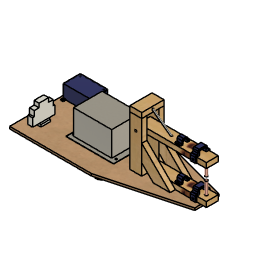
MOT Welder (Autodesk Fusion 360 design; units mm, degrees)
Autodesk Fusion 360 part; units mm, degrees
sketch "Sketch1" plane through (0, 0, 0) normal (0, 0, 1) x (1, 0, 0)
  line L0 (0, 0) -> (600, 0)
  line L1 (600, 0) -> (600, -250)
  line L2 (600, -250) -> (0, -250)
  line L3 (0, -250) -> (0, 0)
  line L4 (300, -250) -> (600, -169.6152)
  line L5 (300, -250) -> (610.5829, -250) construction
  line L6 (300, 0) -> (600, -80.3848)
  dimension "d1" = 600
  dimension "d2" = 250
  dimension "d104" = 15
  dimension "d105" = 15
  constraint horizontal L0
  constraint vertical L1
  constraint horizontal L2
  constraint vertical L3
  constraint coincident L0.start L3.end
  constraint horizontal L5
  constraint midpoint L2 L4.start
  constraint coincident L1 L4.end
  constraint midpoint L0 L6.start
  constraint coincident L1 L6.end
  measures "d1" distance of L1.end L2.end
  measures "d2" distance of L0.start L2.end
  measures "d104" angle of L4 L5
  measures "d105" angle of L0 L6
extrude "Extrude1" add sketch "Sketch1" against normal blind 8 contours L0 L1 L2 L3 L4 L6 makes body 1
sketch "Sketch2" plane through (0, 0, 0) normal (0, 0, 1) x (-1, 0, 0)
  line L0 (0, 250) -> (-300, 250)
  line L1 (-600, 169.6152) -> (-600, 80.3848)
  line L2 (-300, 0) -> (0, 0)
  line L3 (0, 0) -> (0, 250)
  line L4 (0, 0) -> (-150, 0)
  line L5 (-150, 0) -> (-150, 60)
  line L6 (-150, 60) -> (0, 60)
  line L7 (0, 60) -> (0, 0)
  line L8 (-150, 60) -> (-290, 60)
  line L9 (-290, 60) -> (-290, 165)
  line L10 (-290, 165) -> (-150, 165)
  line L11 (-150, 165) -> (-150, 60)
  line L12 (-136, 165) -> (-136, 60)
  line L13 (-290, 179) -> (-150, 179)
  line L14 (-311, 60) -> (-311, 165)
  line L15 (-136, 165) -> (-136, 179)
  line L16 (-136, 179) -> (-150, 179)
  line L17 (-311, 165) -> (-311, 179)
  line L18 (-311, 179) -> (-290, 179)
  line L19 (-311, 60) -> (-290, 60)
  line L20 (-136, 60) -> (-143, 60)
  line L21 (-143, 60) -> (-143, 70)
  line L22 (-143, 70) -> (-136, 70)
  line L23 (-136, 70) -> (-136, 60)
  line L24 (-136, 179) -> (-143, 179)
  line L25 (-143, 179) -> (-143, 159)
  line L26 (-143, 159) -> (-136, 159)
  line L27 (-136, 159) -> (-136, 179)
  line L28 (-311, 60) -> (-300.5, 60)
  line L29 (-300.5, 60) -> (-300.5, 70)
  line L30 (-300.5, 70) -> (-311, 70)
  line L31 (-311, 70) -> (-311, 60)
  line L32 (-311, 179) -> (-300.5, 179)
  line L33 (-300.5, 179) -> (-300.5, 159)
  line L34 (-300.5, 159) -> (-311, 159)
  line L35 (-311, 159) -> (-311, 179)
  circle A0 centre (-143, 70) radius 3
  circle A1 centre (-300.5, 70) radius 3
  circle A2 centre (-300.5, 159) radius 3
  circle A3 centre (-143, 159) radius 3
  line L36 (-300, 250) -> (-600, 169.6152)
  line L37 (-600, 80.3848) -> (-300, 0)
  dimension "d5" = 140
  dimension "d6" = 105
  dimension "d7" = -14
  dimension "d8" = -14
  dimension "d9" = -21
  dimension "d14" = 7
  dimension "d15" = 10
  dimension "d16" = 7
  dimension "d17" = 20
  dimension "d18" = 10
  dimension "d19" = 20
  dimension "d20" = 6
  dimension "d21" = 6
  dimension "d22" = 6
  dimension "d23" = 6
  dimension "d24" = 10.5
  dimension "d25" = 10.5
  dimension "d26" = 150
  dimension "d27" = 60
  constraint horizontal L4
  constraint vertical L5
  constraint horizontal L6
  constraint vertical L7
  constraint coincident L2.end L3.start
  constraint horizontal L8
  constraint vertical L9
  constraint horizontal L10
  constraint vertical L11
  constraint perpendicular L13 L15
  constraint perpendicular L15 L16
  constraint perpendicular L13 L17
  constraint perpendicular L17 L18
  constraint perpendicular L9 L19
  constraint horizontal L20
  constraint vertical L21
  constraint horizontal L22
  constraint vertical L23
  constraint horizontal L24
  constraint vertical L25
  constraint horizontal L26
  constraint vertical L27
  constraint horizontal L28
  constraint vertical L29
  constraint horizontal L30
  constraint vertical L31
  constraint horizontal L32
  constraint vertical L33
  constraint horizontal L34
  constraint vertical L35
  constraint coincident L21.end L22.start
  constraint coincident L29.end L30.start
  constraint coincident L33.end L34.start
  constraint coincident L25.end L26.start
  measures "d5" distance of L5.end L8.end
  measures "d6" distance of L5.end L10.end
  measures "d14" distance of L12.end L20.end
  measures "d15" distance of L12.end L22.end
  measures "d16" distance of L15.end L24.end
  measures "d17" distance of L15.end L26.end
  measures "d18" distance of L14.start L30.end
  measures "d19" distance of L17.end L34.end
  measures "d20" diameter of A0
  measures "d21" diameter of A1
  measures "d22" diameter of A2
  measures "d23" diameter of A3
  measures "d24" distance of L29.end L30.end
  measures "d25" distance of L33.end L34.end
  measures "d26" distance of L5.end L6.end
  measures "d27" distance of L4.end L5.end
extrude "Extrude2" add sketch "Sketch2" along normal blind 1 separate body contours L6 L12 L20 L21 L22 L23 A0 | L6 L9 L10 L11 L12 L13 L14 L16 L18 L19 L21 L22 L25 L26 L29 L30 L33 L34 A0 A1 A2 A3 | L12 L15 L16 L24 L25 L26 L27 A3 | L14 L19 L28 L29 L30 L31 A1 | L14 L17 L18 L32 L33 L34 L35 A2 makes body 2
extrude "Extrude3" add sketch "Sketch2" along normal blind 92 separate body contours L8 L9 L10 L11 makes body 3
combine "Combine2" operation add target body 3 tool bodies 2
ref_plane "WorkPlane1" through (370, -112.5, 46) normal (1, 0, 0) x (0, 1, 0)
sketch "Sketch3" plane through (370, 0, 0) normal (1, 0, 0) x (0, 1, 0)
  line L0 (0, 0) -> (-250, 0)
  line L1 (-125, 0) -> (-125, 9.5)
  line L2 (-103, 0) -> (-147, 0)
  line L3 (-147, 0) -> (-147, 19)
  line L4 (-147, 19) -> (-103, 19)
  line L5 (-103, 19) -> (-103, 0)
  line L6 (-103, 0) -> (-147, 19) construction
  line L7 (-147, 0) -> (-103, 19) construction
  line L8 (-125, 19) -> (-125, 124)
  line L9 (-125, 124) -> (-125, 133.5)
  line L10 (-103, 124) -> (-147, 124)
  line L11 (-147, 124) -> (-147, 143)
  line L12 (-147, 143) -> (-103, 143)
  line L13 (-103, 143) -> (-103, 124)
  line L14 (-103, 124) -> (-147, 143) construction
  line L15 (-147, 124) -> (-103, 143) construction
  point P0 (-125, 9.5)
  point P1 (-125, 133.5)
  dimension "d29" = 250
  dimension "d30" = 9.5
  dimension "d31" = 44
  dimension "d32" = 105
  dimension "d33" = 9.5
  dimension "d34" = 44
  dimension "d35" = 19
  constraint coincident L0.start origin
  constraint horizontal L0
  constraint midpoint L0 L1.start
  constraint perpendicular L0 L1
  constraint horizontal L2
  constraint perpendicular L2 L3
  constraint parallel L2 L4
  constraint parallel L3 L5
  constraint coincident L6 P0
  constraint coincident L7 P0
  constraint coincident P0 L1.end
  constraint midpoint L4 L8.start
  constraint perpendicular L4 L8
  constraint vertical L9
  constraint horizontal L10
  constraint perpendicular L10 L11
  constraint parallel L10 L12
  constraint parallel L11 L13
  constraint coincident L14 P1
  constraint coincident L15 P1
  constraint coincident P1 L9.end
  measures "d29" distance of L0.start L0.end
  measures "d30" distance of L1.start P0
  measures "d31" distance of L3.end L4.end
  measures "d32" distance of L8.start L8.end
  measures "d33" distance of L8.end P1
  measures "d34" distance of L11.end L12.end
  measures "d35" distance of L10.end L11.end
extrude "Extrude4" add sketch "Sketch3" along normal blind 250 separate body makes body 4 at (453.3333, -117.6667, 124) makes body 5 at (453.3333, -117.6667, 0)
sketch "Sketch5" plane through (0, -103, 0) normal (0, 1, 0) x (-1, 0, 0)
  line L0 (-370, 124) -> (-370, 143)
  line L1 (-370, 143) -> (-620, 143)
  line L2 (-620, 143) -> (-620, 124)
  line L3 (-620, 124) -> (-370, 124)
  line L4 (-370, 124) -> (-379.5, 124)
  line L5 (-379.5, 124) -> (-379.5, 133.5)
  line L6 (-379.5, 133.5) -> (-370, 133.5)
  line L7 (-370, 133.5) -> (-370, 124)
  circle A0 centre (-379.5, 133.5) radius 4
  circle A1 centre (-379.5, 133.5) radius 11
  line L8 (-357.5, 183.5) -> (-401.5, 183.5)
  line L9 (-401.5, 183.5) -> (-401.5, 83.5)
  line L10 (-401.5, 83.5) -> (-357.5, 83.5)
  line L11 (-357.5, 83.5) -> (-357.5, 183.5)
  line L12 (-357.5, 183.5) -> (-401.5, 83.5) construction
  line L13 (-401.5, 183.5) -> (-357.5, 83.5) construction
  line L14 (-401.5, 83.5) -> (-357.5, 83.5)
  line L15 (-357.5, 83.5) -> (-357.5, 0)
  line L16 (-357.5, 0) -> (-401.5, 0)
  line L17 (-401.5, 0) -> (-401.5, 83.5)
  line L18 (-401.5, 0) -> (-422.7132, 21.2132)
  line L19 (-401.5, 0) -> (-357.5, 0) construction
  line L20 (-422.7132, 21.2132) -> (-401.5, 42.4264)
  line L21 (-422.7132, 21.2132) -> (-443.9264, 0)
  line L22 (-401.5, 0) -> (-443.9264, 0)
  line L23 (-453.8259, 52.3259) -> (-475.0391, 31.1127)
  line L24 (-453.8259, 52.3259) -> (-432.6127, 73.5391)
  line L25 (-443.9264, 0) -> (-506.1518, 0)
  line L26 (-506.1518, 0) -> (-475.0391, 31.1127)
  line L27 (-432.6127, 73.5391) -> (-401.5, 104.6518)
  point P0 (-379.5, 133.5)
  dimension "d38" = 9.5
  dimension "d39" = 9.5
  dimension "d40" = 8
  dimension "d41" = 22
  dimension "d42" = 44
  dimension "d43" = 100
  dimension "d44" = 44
  dimension "d45" = 83.5
  dimension "d57" = 135
  dimension "d58" = 30
  dimension "d59" = -44
  constraint horizontal L4
  constraint vertical L5
  constraint horizontal L6
  constraint vertical L7
  constraint coincident L0.start L3.end
  constraint coincident P0 L5.end
  constraint concentric A0 A1
  constraint horizontal L8
  constraint perpendicular L8 L9
  constraint parallel L8 L10
  constraint parallel L9 L11
  constraint coincident L12 P0
  constraint coincident L13 P0
  constraint horizontal L14
  constraint vertical L15
  constraint horizontal L16
  constraint vertical L17
  constraint horizontal L19
  constraint coincident L17 L20.end
  constraint perpendicular L18 L20
  constraint perpendicular L18 L21
  constraint perpendicular L17 L22
  constraint parallel L22 L25
  constraint parallel L23 L26
  constraint coincident L17 L27.end
  constraint parallel L24 L27
  measures "d38" distance of L0.start L4.end
  measures "d39" distance of L0.start L6.end
  measures "d40" diameter of A0
  measures "d41" diameter of A1
  measures "d42" distance of L9.end L10.end
  measures "d43" distance of L8.end L9.end
  measures "d44" distance of L9.end L10.end
  measures "d45" distance of L9.end L16.end
  measures "d57" angle of L18 L19
  measures "d58" distance of L16.end L18.end
extrude "Extrude5" add sketch "Sketch5" along normal blind 19 separate body contours L0 L3 L4 L7 A1 | L0 L1 L3 L4 L7 A1 L8 L9 L10 L11 L14 | L0 L3 L4 L5 L6 L7 A0 A1 | L0 L7 A1 | L3 L4 A1 | L0 L1 L3 L5 L6 A0 A1 | L1 L3 A1 L9 | L0 L1 A1 | L1 A1 | L10 L14 L15 L16 L17 makes body 6
extrude "Extrude6" cut sketch "Sketch5" along normal blind 7 contours L0 L3 L4 L5 L6 L7 A0 A1 | L0 L7 A1 | L3 L4 A1 | L0 L1 L3 L5 L6 A0 A1 | L1 A1 bodies 6
extrude "Extrude8" add sketch "Sketch5" along normal blind 19 separate body contours L9 L17 L20 L21 L23 L24 L25 L26 L27 makes body 7
ref_plane "WorkPlane2" through (495, -125, 133.5) normal (0, 1, 0) x (0, 0, 1)
mirror "Mirror1" about plane through (495, -125, 133.5) normal (0, 1, 0) of bodies 7 6 makes body 8 at (379.4004, -166, 43.1704) makes body 9 at (475.0391, -147, 10.3709)
sketch "Sketch6" plane through (0, 0, 183.5) normal (0, 0, 1) x (-1, 0, 0)
  line L0 (-357.5, 103) -> (-401.5, 103)
  line L1 (-401.5, 103) -> (-401.5, 84)
  line L2 (-401.5, 84) -> (-357.5, 84)
  line L3 (-357.5, 84) -> (-357.5, 103)
  line L4 (-357.5, 84) -> (-401.5, 84)
  line L5 (-401.5, 84) -> (-401.5, 166)
  line L6 (-401.5, 166) -> (-357.5, 166)
  line L7 (-357.5, 166) -> (-357.5, 84)
  dimension "d53" = 44
  dimension "d54" = 82
  constraint horizontal L4
  constraint vertical L5
  constraint horizontal L6
  constraint vertical L7
  constraint coincident L2.end L3.start
  measures "d53" distance of L2.end L1.end
  measures "d54" distance of L2.end L6.end
extrude "Extrude7" add sketch "Sketch6" along normal blind 19 separate body makes body 10
sketch "Sketch7" plane through (0, 0, -8) normal (0, 0, -1) x (1, 0, 0)
  line L0 (300, 250) -> (0, 250)
  line L1 (0, 250) -> (0, 0)
  line L2 (0, 0) -> (300, 0)
  line L3 (600, 80.3848) -> (600, 169.6152)
  line L4 (0, 250) -> (40, 250)
  line L5 (40, 250) -> (40, 210)
  line L6 (40, 210) -> (0, 210)
  line L7 (0, 210) -> (0, 250)
  circle A0 centre (40, 210) radius 21.5
  circle A1 centre (40, 210) radius 29
  line L8 (600, 169.6152) -> (300, 250)
  line L9 (300, 0) -> (600, 80.3848)
  dimension "d62" = 40
  dimension "d63" = 40
  dimension "d64" = 43
  dimension "d65" = 58
  constraint horizontal L4
  constraint vertical L5
  constraint horizontal L6
  constraint vertical L7
  constraint coincident L0.end L1.start
  constraint coincident L5.end L6.start
  constraint concentric A0 A1
  measures "d62" distance of L0.end L4.end
  measures "d63" distance of L0.end L6.end
  measures "d64" diameter of A0
  measures "d65" diameter of A1
extrude "Extrude9" add sketch "Sketch7" along normal blind 20 separate body contours L5 L6 A0 | L5 L6 A0 makes body 11
loft "Loft1" add profiles "Sketch7" section 1 contours L5 L6 A0 A1 | L5 L6 A0 A1 section 2 face at (46.6953, -203.71, -28) separate body on bodies 11 makes body 12
combine "Combine1" operation add target body 11 tool bodies 12
fillet "Fillet1" radius 5 1 edges at (19.955, -202.2253, -28) on bodies 11
pattern_linear "R-Pattern1" count 2 spacing 170 along (0, 1, 0) count 2 spacing 260 along (1, 0, 0) of bodies 11 makes body 13 at (44.1141, -67.2954, -11.7235) makes body 14 at (304.1141, -237.2954, -11.7235) makes body 15 at (304.1141, -67.2954, -11.7235)
sketch "Sketch8" plane through (0, 0, 124) normal (0, 0, -1) x (1, 0, 0)
  line L0 (370, 147) -> (370, 103)
  line L1 (370, 103) -> (620, 103)
  line L2 (620, 103) -> (620, 147)
  line L3 (620, 147) -> (370, 147)
  line L4 (620, 147) -> (598, 147)
  line L5 (598, 147) -> (598, 125)
  line L6 (598, 125) -> (620, 125)
  line L7 (620, 125) -> (620, 147)
  circle A0 centre (598, 125) radius 5
  dimension "d74" = 22
  dimension "d75" = 10
  constraint horizontal L4
  constraint vertical L5
  constraint horizontal L6
  constraint vertical L7
  constraint coincident L2.end L3.start
  constraint coincident L5.end L6.start
  measures "d74" distance of L2.end L4.end
  measures "d75" diameter of A0
extrude "Extrude10" add sketch "Sketch8" along normal blind 105 separate body contours L5 L6 A0 | L5 L6 A0 makes body 16
extrude "Extrude11" cut 1 faces at (599.0448, -126.4407, 124) along direction (0, 0, -1) blind 54.5 on bodies 16 bodies 16
extrude "Extrude12" add sketch "Sketch8" along normal blind 50.5 separate body contours L5 L6 A0 | L5 L6 A0 makes body 17
chamfer "Chamfer1" distance 5 angle 45 2 edges at (593.3384, -123.1919, 69.5) (593.3384, -123.1919, 73.5) on bodies 16 17
sketch "Sketch9" plane through (401.5, 0, 0) normal (1, 0, 0) x (0, 1, 0)
  line L0 (-166, 183.5) -> (-84, 183.5)
  line L1 (-84, 183.5) -> (-84, 202.5)
  line L2 (-84, 202.5) -> (-166, 202.5)
  line L3 (-166, 202.5) -> (-166, 183.5)
  line L4 (-125, 202.5) -> (-125, 193)
  circle A0 centre (-125, 193) radius 3.5
  dimension "d83" = 9.5
  dimension "d84" = 7
  constraint midpoint L2 L4.start
  constraint perpendicular L2 L4
  constraint coincident L4.end A0.centre
  measures "d83" distance of L4.start L4.end
  measures "d84" diameter of A0
sketch "Sketch10" plane through (0, 0, 143) normal (0, 0, 1) x (-1, 0, 0)
  line L0 (-370, 103) -> (-370, 147)
  line L1 (-370, 147) -> (-620, 147)
  line L2 (-620, 147) -> (-620, 103)
  line L3 (-620, 103) -> (-370, 103)
  line L4 (-370, 125) -> (-470, 125)
  circle A0 centre (-470, 125) radius 3.5
  dimension "d85" = 100
  dimension "d86" = 7
  constraint midpoint L0 L4.start
  constraint perpendicular L0 L4
  constraint coincident L4.end A0.centre
  measures "d85" distance of L4.start L4.end
  measures "d86" diameter of A0
loft "Loft2" add profiles "Sketch10", "Sketch9" section 1 contours A0 section 2 contours A0 separate body makes body 18
sketch "Sketch11" plane through (0, 0, 0) normal (0, 0, 1) x (-1, 0, 0)
  line L0 (0, 250) -> (-300, 250)
  line L1 (-600, 169.6152) -> (-600, 80.3848)
  line L2 (-300, 0) -> (0, 0)
  line L3 (0, 0) -> (0, 250)
  line L4 (0, 0) -> (-30, 0)
  line L5 (-30, 0) -> (-30, 160)
  line L6 (-30, 160) -> (0, 160)
  line L7 (0, 160) -> (0, 0)
  line L8 (-30, 160) -> (-60, 160)
  line L9 (-60, 160) -> (-60, 195)
  line L10 (-60, 195) -> (-30, 195)
  line L11 (-30, 195) -> (-30, 160)
  line L12 (-300, 250) -> (-600, 169.6152)
  line L13 (-600, 80.3848) -> (-300, 0)
  dimension "d87" = 30
  dimension "d88" = 160
  dimension "d89" = 30
  dimension "d90" = 35
  constraint horizontal L4
  constraint vertical L5
  constraint horizontal L6
  constraint vertical L7
  constraint coincident L2.end L3.start
  constraint horizontal L8
  constraint vertical L9
  constraint horizontal L10
  constraint vertical L11
  measures "d87" distance of L2.end L4.end
  measures "d88" distance of L2.end L6.end
  measures "d89" distance of L5.end L8.end
  measures "d90" distance of L5.end L10.end
extrude "Extrude13" add sketch "Sketch11" along normal blind 8 separate body contours L8 L9 L10 L11 makes body 19
sketch "Sketch12" plane through (0, 0, 8) normal (0, 0, 1) x (-1, 0, 0)
  line L0 (-30, 195) -> (-60, 195)
  line L1 (-60, 195) -> (-60, 160)
  line L2 (-60, 160) -> (-30, 160)
  line L3 (-30, 160) -> (-30, 195)
  line L4 (-53.2298, 136.6132) -> (-35.2298, 136.6132)
  line L5 (-35.2298, 136.6132) -> (-35.2298, 218.6132)
  line L6 (-35.2298, 218.6132) -> (-53.2298, 218.6132)
  line L7 (-53.2298, 218.6132) -> (-53.2298, 136.6132)
  line L8 (-53.2298, 136.6132) -> (-35.2298, 218.6132) construction
  line L9 (-35.2298, 136.6132) -> (-53.2298, 218.6132) construction
  line L10 (-35.2298, 212.6132) -> (-53.2298, 212.6132)
  line L11 (-53.2298, 212.6132) -> (-53.2298, 142.6132)
  line L12 (-53.2298, 142.6132) -> (-35.2298, 142.6132)
  line L13 (-35.2298, 142.6132) -> (-35.2298, 212.6132)
  line L14 (-35.2298, 212.6132) -> (-53.2298, 142.6132) construction
  line L15 (-53.2298, 212.6132) -> (-35.2298, 142.6132) construction
  line L16 (-47.674, 155.1132) -> (-40.7856, 155.1132)
  line L17 (-40.7856, 155.1132) -> (-40.7856, 200.1132)
  line L18 (-40.7856, 200.1132) -> (-47.674, 200.1132)
  line L19 (-47.674, 200.1132) -> (-47.674, 155.1132)
  line L20 (-47.674, 155.1132) -> (-40.7856, 200.1132) construction
  line L21 (-40.7856, 155.1132) -> (-47.674, 200.1132) construction
  point P0 (-44.2298, 177.6132)
  point P1 (-44.2298, 177.6132)
  point P2 (-44.2298, 177.6132)
  dimension "d93" = 18
  dimension "d94" = 82
  dimension "d95" = 18
  dimension "d96" = 70
  dimension "d97" = 45
  constraint horizontal L4
  constraint perpendicular L4 L5
  constraint parallel L4 L6
  constraint parallel L5 L7
  constraint coincident L8 P2
  constraint coincident L9 P2
  constraint horizontal L10
  constraint perpendicular L10 L11
  constraint parallel L10 L12
  constraint parallel L11 L13
  constraint coincident L14 P2
  constraint coincident L15 P2
  constraint coincident P2 P1
  constraint horizontal L16
  constraint perpendicular L16 L17
  constraint parallel L16 L18
  constraint parallel L17 L19
  constraint coincident L20 P2
  constraint coincident L21 P2
  measures "d93" distance of L5.end L6.end
  measures "d94" distance of L4.end L5.end
  measures "d95" distance of L11.end L12.end
  measures "d96" distance of L10.end L11.end
  measures "d97" distance of L16.end L17.end
extrude "Extrude14" add sketch "Sketch12" along normal blind 65 separate body contours L0 L2 L5 L13 L17 | L0 L2 L17 L19 | L0 L2 L7 L11 L19 makes body 20
extrude "Extrude15" add sketch "Sketch12" along normal blind 50 contours L0 L5 L7 L10 L11 L13 L17 L18 L19 | L0 L17 L18 L19 | L2 L5 L7 L11 L12 L13 L16 L17 L19 | L2 L16 L17 L19 bodies 19 20
extrude "Extrude16" add sketch "Sketch12" along normal blind 30 contours L5 L6 L7 L10 | L4 L5 L7 L12 bodies 19
copy_body "CopyPasteBodies1" bodies 14 makes body 21
move_body "Move1" bodies 21 to x (1, 0, 0) y (0, 1, 0) z (0, 0, 1) at (260, 85, 0)
sketch "Sketch14" plane through (0, 0, 0) normal (0, 0, 1) x (-1, 0, 0)
  line L0 (-300, 250) -> (-600, 169.6152)
  line L1 (-600, 169.6152) -> (-600, 80.3848)
  line L2 (-600, 80.3848) -> (-300, 0)
  line L3 (-300, 0) -> (0, 0)
  line L4 (0, 0) -> (0, 250)
  line L5 (0, 250) -> (-300, 250)
  line L6 (0, 0) -> (-100, 0)
  line L7 (-100, 0) -> (-100, 3)
  line L8 (-100, 3) -> (0, 3)
  line L9 (0, 3) -> (0, 0)
  line L10 (0, 0) -> (-3, 0)
  line L11 (-3, 0) -> (-3, 60)
  line L12 (-3, 60) -> (0, 60)
  line L13 (0, 60) -> (0, 0)
  line L14 (-100, 0) -> (-97, 0)
  line L15 (-97, 0) -> (-97, 60)
  line L16 (-97, 60) -> (-100, 60)
  line L17 (-100, 60) -> (-100, 0)
  line L18 (-3, 60) -> (0, 60)
  line L19 (0, 60) -> (-3, 60)
  line L20 (-87, 250) -> (-90, 250)
  line L21 (-97, 3) -> (-89, 3)
  line L22 (-89, 3) -> (-89, 11)
  line L23 (-89, 11) -> (-97, 11)
  line L24 (-97, 11) -> (-97, 3)
  line L25 (-3, 3) -> (-11, 3)
  line L26 (-11, 3) -> (-11, 11)
  line L27 (-11, 11) -> (-3, 11)
  line L28 (-3, 11) -> (-3, 3)
  line L29 (-97, 3) -> (-89, 11)
  line L30 (-11, 11) -> (-3, 3)
  circle A0 centre (-93, 7) radius 2.25
  circle A1 centre (-7, 7) radius 2.25
  line L31 (-100, 0) -> (-110, 0)
  line L32 (-110, 0) -> (-110, 10)
  line L33 (-110, 10) -> (-100, 10)
  line L34 (-100, 10) -> (-100, 0)
  line L35 (0, 0) -> (10, 0)
  line L36 (10, 0) -> (10, 10)
  line L37 (10, 10) -> (0, 10)
  line L38 (0, 10) -> (0, 0)
  circle A2 centre (-105, 5) radius 1.7
  circle A3 centre (5, 5) radius 1.7
  line L39 (-90, 250) -> (-100, 250)
  line L40 (-100, 60) -> (0, 60)
  line L41 (0, 60) -> (0, 63)
  line L42 (0, 63) -> (-100, 63)
  line L43 (-100, 63) -> (-100, 60)
  line L44 (0, 63) -> (-10, 63)
  line L45 (-10, 63) -> (-10, 73)
  line L46 (-10, 73) -> (0, 73)
  line L47 (0, 73) -> (0, 63)
  line L48 (-100, 63) -> (-90, 63)
  line L49 (-90, 63) -> (-90, 73)
  line L50 (-90, 73) -> (-100, 73)
  line L51 (-100, 73) -> (-100, 63)
  circle A4 centre (-5, 68) radius 1.7
  circle A5 centre (-95, 68) radius 1.7
  dimension "d112" = 100
  dimension "d113" = 3
  dimension "d116" = 3
  dimension "d117" = 60
  dimension "d118" = 3
  dimension "d119" = 60
  dimension "d191" = 3
  dimension "d200" = 8
  dimension "d201" = 8
  dimension "d202" = 8
  dimension "d203" = 8
  dimension "d204" = 4.5
  dimension "d205" = 4.5
  dimension "d223" = 10
  dimension "d224" = 10
  dimension "d225" = 10
  dimension "d226" = 10
  dimension "d227" = 3.4
  dimension "d228" = 3.4
  dimension "d240" = 3
  dimension "d254" = 10
  dimension "d255" = 10
  dimension "d256" = 10
  dimension "d257" = 10
  dimension "d258" = 3.4
  dimension "d259" = 3.4
  constraint horizontal L6
  constraint vertical L7
  constraint horizontal L8
  constraint vertical L9
  constraint coincident L3.end L4.start
  constraint horizontal L10
  constraint vertical L11
  constraint horizontal L12
  constraint vertical L13
  constraint horizontal L14
  constraint vertical L15
  constraint horizontal L16
  constraint vertical L17
  constraint horizontal L18
  constraint horizontal L19
  constraint horizontal L20
  constraint horizontal L21
  constraint vertical L22
  constraint horizontal L23
  constraint vertical L24
  constraint coincident L15 L21.start
  constraint coincident L8 L21.start
  constraint horizontal L25
  constraint vertical L26
  constraint horizontal L27
  constraint vertical L28
  constraint coincident L11 L25.start
  constraint coincident L8 L25.start
  constraint midpoint L29 A0.centre
  constraint midpoint L30 A1.centre
  constraint horizontal L31
  constraint vertical L32
  constraint horizontal L33
  constraint vertical L34
  constraint horizontal L35
  constraint vertical L36
  constraint horizontal L37
  constraint vertical L38
  constraint horizontal L39
  constraint horizontal L40
  constraint vertical L41
  constraint horizontal L42
  constraint vertical L43
  constraint coincident L4 L41.end
  constraint horizontal L44
  constraint vertical L45
  constraint horizontal L46
  constraint vertical L47
  constraint horizontal L48
  constraint vertical L49
  constraint horizontal L50
  constraint vertical L51
  measures "d112" distance of L3.end L6.end
  measures "d113" distance of L3.end L8.end
  measures "d116" distance of L3.end L10.end
  measures "d117" distance of L3.end L12.end
  measures "d118" distance of L6.end L14.end
  measures "d119" distance of L6.end L16.end
  measures "d191" distance of L20.start L20.end
  measures "d200" distance of L21.start L21.end
  measures "d201" distance of L21.start L23.end
  measures "d202" distance of L25.start L25.end
  measures "d203" distance of L25.start L27.end
  measures "d204" diameter of A0
  measures "d205" diameter of A1
  measures "d223" distance of L6.end L31.end
  measures "d224" distance of L6.end L33.end
  measures "d225" distance of L3.end L35.end
  measures "d226" distance of L3.end L37.end
  measures "d227" diameter of A2
  measures "d228" diameter of A3
  measures "d240" distance of L16.end L42.end
  measures "d254" distance of L41.end L44.end
  measures "d255" distance of L41.end L46.end
  measures "d256" distance of L42.end L48.end
  measures "d257" distance of L42.end L50.end
  measures "d258" diameter of A4
  measures "d259" diameter of A5
extrude "Extrude19" add sketch "Sketch14" along normal blind 45 separate body contours L3 L6 L7 L8 L14 L15 L17 L34 | L3 L6 L8 L11 L15 L21 L25 | L8 L15 L16 L17 L24 L34 L40 | L3 L4 L6 L8 L9 L10 L11 L13 L38 | L8 L21 L22 L29 A0 | L15 L23 L24 L29 A0 | L4 L8 L11 L12 L13 L18 L19 L28 L38 L40 | L11 L27 L28 L30 A1 | L8 L25 L26 L30 A1 makes body 22
extrude "Extrude32" cut sketch "Sketch14" along normal blind 38 contours L8 L21 L22 L29 A0 | L15 L23 L24 L29 A0 | L11 L27 L28 L30 A1 | L8 L25 L26 L30 A1 bodies 22
ref_plane "WorkPlane3" through (585, -125, 9.5) normal (1, 0, 0) x (0, 0, -1)
sketch "Sketch15" plane through (585, 0, 0) normal (1, 0, 0) x (0, 1, 0)
  line L0 (0, 0) -> (-103, 0)
  line L1 (-103, 0) -> (-103, 19)
  line L2 (-103, 19) -> (-103, 24)
  line L3 (-103, 19) -> (-125, 19)
  line L4 (-125, 19) -> (-125, 26.5)
  line L5 (-113, 19) -> (-137, 19)
  line L6 (-137, 19) -> (-137, 34)
  line L7 (-137, 34) -> (-113, 34)
  line L8 (-113, 34) -> (-113, 19)
  line L9 (-113, 19) -> (-137, 34) construction
  line L10 (-137, 19) -> (-113, 34) construction
  line L11 (-137, 19) -> (-147, 19)
  line L12 (-147, 19) -> (-147, 24)
  line L13 (-147, 24) -> (-137, 24)
  line L14 (-113, 24) -> (-103, 24)
  line L15 (-142, 14) -> (-142, 39)
  line L16 (-142, 39) -> (-108, 39)
  line L17 (-108, 39) -> (-108, 14)
  line L18 (-108, 14) -> (-142, 14)
  line L19 (-103, 24) -> (-98, 24)
  line L20 (-98, 24) -> (-98, 0)
  line L21 (-98, 0) -> (-103, 0)
  line L22 (-103, 0) -> (-103, 24)
  line L23 (-147, 24) -> (-152, 24)
  line L24 (-152, 24) -> (-152, 0)
  line L25 (-152, 0) -> (-147, 0)
  line L26 (-147, 0) -> (-147, 24)
  point P0 (-125, 26.5)
  dimension "d129" = 103
  dimension "d130" = 19
  dimension "d131" = 5
  dimension "d132" = 22
  dimension "d133" = 7.5
  dimension "d134" = 24
  dimension "d135" = 10
  dimension "d136" = 5
  dimension "d137" = -5
  dimension "d138" = 5
  dimension "d139" = 5
  dimension "d174" = 15
  constraint coincident L0.start origin
  constraint horizontal L0
  constraint perpendicular L0 L1
  constraint perpendicular L0 L2
  constraint perpendicular L2 L3
  constraint perpendicular L3 L4
  constraint horizontal L5
  constraint perpendicular L5 L6
  constraint parallel L5 L7
  constraint parallel L6 L8
  constraint coincident L9 P0
  constraint coincident L10 P0
  constraint coincident P0 L4.end
  constraint perpendicular L6 L11
  constraint perpendicular L11 L12
  constraint coincident L6 L13.end
  constraint perpendicular L6 L13
  constraint coincident L8 L14.start
  constraint perpendicular L8 L14
  constraint horizontal L19
  constraint vertical L20
  constraint horizontal L21
  constraint vertical L22
  constraint horizontal L23
  constraint vertical L24
  constraint horizontal L25
  constraint vertical L26
  measures "d129" distance of L0.start L0.end
  measures "d130" distance of L0.end L1.end
  measures "d131" distance of L1.end L2.end
  measures "d132" distance of L1.end L3.end
  measures "d133" distance of L3.end P0
  measures "d134" distance of L6.end L7.end
  measures "d135" distance of L5.end L11.end
  measures "d136" distance of L11.end L12.end
  measures "d138" distance of L2.end L19.end
  measures "d139" distance of L12.end L23.end
  measures "d174" distance of L5.end L6.end
extrude "Extrude21" add sketch "Sketch15" against normal blind 20 separate body contours L0 L1 L2 L19 L20 L21 L22 | L2 L3 L14 L17 L22 | L3 L8 L14 L17 | L6 L7 L8 L13 L14 L15 L16 L17 | L6 L11 L13 L15 | L11 L12 L13 L15 L26 | L12 L23 L24 L25 L26 makes body 23
chamfer "Chamfer3" distance 4 angle 45 6 edges at (575, -142, 24) (575, -108, 24) (575, -108, 39) (575, -142, 39) (575, -152, 24) (575, -98, 24) on bodies 23
sketch "Sketch16" plane through (0, -152, 0) normal (0, -1, 0) x (1, 0, 0)
  line L0 (585, 0) -> (585, 20)
  line L1 (565, 20) -> (565, 0)
  line L2 (565, 0) -> (585, 0)
  line L3 (585, 0) -> (575, 0)
  line L4 (575, 0) -> (575, 9.5)
  line L5 (575, 9.5) -> (585, 9.5)
  line L6 (585, 9.5) -> (585, 0)
  circle A0 centre (575, 9.5) radius 1.7
  line L7 (585, 20) -> (565, 20)
  dimension "d143" = 10
  dimension "d144" = 9.5
  dimension "d145" = 3.4
  constraint horizontal L3
  constraint vertical L4
  constraint horizontal L5
  constraint vertical L6
  constraint coincident L0.start L2.end
  constraint coincident L4.end L5.start
  measures "d143" distance of L0.start L3.end
  measures "d144" distance of L0.start L5.end
  measures "d145" diameter of A0
extrude "Extrude22" cut sketch "Sketch16" against normal blind 54 contours L4 L5 A0 | L4 L5 A0 bodies 5 23
ref_plane "WorkPlane4" through (520, -125, 9.5) normal (1, 0, 0) x (0, 0, -1)
sketch "Sketch17" plane through (520, 0, 0) normal (1, 0, 0) x (0, 1, 0)
  line L0 (0, 0) -> (-125, 0)
  line L1 (-125, 0) -> (-125, 19)
  line L2 (-125, 19) -> (-125, 34)
  line L3 (-125, 34) -> (-117.5, 34)
  line L4 (-117.5, 34) -> (-117.5, 19)
  line L5 (-117.5, 19) -> (-107.5, 19)
  line L6 (-107.5, 19) -> (-107.5, 22)
  line L7 (-107.5, 22) -> (-114.5, 22)
  line L8 (-114.5, 22) -> (-114.5, 37)
  line L9 (-125, 34) -> (-125, 37)
  line L10 (-125, 37) -> (-114.5, 37)
  dimension "d149" = 125
  dimension "d150" = 19
  dimension "d151" = 15
  dimension "d153" = 7.5
  dimension "d154" = 10
  dimension "d155" = 3
  dimension "d156" = 7
  dimension "d157" = 15
  dimension "d158" = 15
  dimension "d159" = 3
  constraint coincident L0.start origin
  constraint horizontal L0
  constraint perpendicular L0 L1
  constraint parallel L1 L2
  constraint perpendicular L2 L3
  constraint perpendicular L3 L4
  constraint perpendicular L4 L5
  constraint perpendicular L5 L6
  constraint perpendicular L4 L7
  constraint perpendicular L3 L8
  constraint perpendicular L3 L9
  measures "d149" distance of L0.start L0.end
  measures "d150" distance of L0.end L1.end
  measures "d151" distance of L1.end L2.end
  measures "d153" distance of L2.end L3.end
  measures "d154" distance of L4.end L5.end
  measures "d155" distance of L5.end L6.end
  measures "d156" distance of L6.end L7.end
  measures "d157" distance of L7.end L8.end
  measures "d158" distance of L3.end L4.end
  measures "d159" distance of L2.end L9.end
extrude "Extrude23" add sketch "Sketch17" against normal blind 20 separate body makes body 24
fillet "Fillet2" radius 7.5 1 edges at (510, -117.5, 34) on bodies 24
chamfer "Chamfer4" distance 5 angle 45 1 edges at (510, -114.5, 37) on bodies 24
sketch "Sketch18" plane through (0, 0, 22) normal (0, 0, 1) x (-1, 0, 0)
  line L0 (-520, 114.5) -> (-520, 107.5)
  line L1 (-520, 107.5) -> (-500, 107.5)
  line L2 (-500, 107.5) -> (-500, 114.5)
  line L3 (-500, 114.5) -> (-520, 114.5)
  line L4 (-520, 111) -> (-510, 111)
  circle A0 centre (-510, 111) radius 1.7
  dimension "d165" = 3.4
  constraint midpoint L0 L4.start
  constraint perpendicular L2 L4
  constraint coincident L4.end A0.centre
  measures "d165" diameter of A0
extrude "Extrude24" cut sketch "Sketch18" against normal blind 3 contours A0 bodies 24
chamfer "Chamfer5" distance 1.7 angle 45 1 edges at (511.585, -111.6147, 22) on bodies 24
mirror "Mirror2" about plane through (520, -125, 34) normal (0, -1, 0) of bodies 24 merged
chamfer "Chamfer6" distance 1.7 angle 45 2 edges at (573.415, -152, 10.1147) (573.415, -98, 8.8853) on bodies 23
chamfer "Chamfer7" distance 1 angle 45 10 edges at (520, -135.5, 27) (520, -133, 34.5) (520, -125, 37) (520, -117, 34.5) (520, -114.5, 27) (500, -135.5, 27) (500, -133, 34.5) (500, -125, 37) (500, -114.5, 27) (500, -117, 34.5) on bodies 24
chamfer "Chamfer8" distance 1 angle 45 28 edges at (585, -152, 10) (585, -150, 22) (585, -147, 24) (585, -144, 26) (585, -142, 31.5) (585, -140, 37) (585, -125, 39) (565, -125, 39) (565, -140, 37) (565, -142, 31.5) (565, -144, 26) (565, -147, 24) (565, -150, 22) (565, -152, 10) (575, -152, 0) (585, -110, 37) (585, -108, 31.5) (585, -106, 26) (585, -103, 24) (585, -100, 22) (565, -110, 37) (565, -108, 31.5) (565, -100, 22) (565, -103, 24) (565, -106, 26) (565, -98, 10) (585, -98, 10) (575, -98, 0) on bodies 23
copy_body "CopyPasteBodies2" bodies 23 makes body 25
copy_body "CopyPasteBodies3" bodies 24 makes body 26
move_body "Move2" bodies 26 23 to x (1, 0, 0) y (0, 1, 0) z (0, 0, 1) at (0, 0, 124)
sketch "Sketch19" plane through (0, 0, 0) normal (0, 1, 0) x (-1, 0, 0)
  line L0 (-100, 0) -> (0, 0)
  line L1 (0, 0) -> (0, 45)
  line L2 (0, 45) -> (-100, 45)
  line L3 (-100, 45) -> (-100, 0)
  line L4 (0, 0) -> (-20, 0)
  line L5 (-20, 0) -> (-20, 10)
  line L6 (-20, 10) -> (0, 10)
  line L7 (0, 10) -> (0, 0)
  line L8 (-20, 10) -> (-47.5, 10)
  line L9 (-47.5, 10) -> (-47.5, 30)
  line L10 (-47.5, 30) -> (-20, 30)
  line L11 (-20, 30) -> (-20, 10)
  line L12 (-20, 20) -> (-13, 20)
  circle A0 centre (-13, 20) radius 2.25
  line L13 (-47.5, 20) -> (-54.5, 20)
  circle A1 centre (-54.5, 20) radius 1.75
  line L14 (-50.5, 24) -> (-58.5, 24)
  line L15 (-58.5, 24) -> (-58.5, 16)
  line L16 (-58.5, 16) -> (-50.5, 16)
  line L17 (-50.5, 16) -> (-50.5, 24)
  line L18 (-50.5, 24) -> (-58.5, 16) construction
  line L19 (-58.5, 24) -> (-50.5, 16) construction
  line L20 (-9, 24) -> (-17, 24)
  line L21 (-17, 24) -> (-17, 16)
  line L22 (-17, 16) -> (-9, 16)
  line L23 (-9, 16) -> (-9, 24)
  line L24 (-9, 24) -> (-17, 16) construction
  line L25 (-17, 24) -> (-9, 16) construction
  line L26 (-54.5, 20) -> (-79.5, 20)
  line L27 (-68.5, 35) -> (-90.5, 35)
  line L28 (-90.5, 35) -> (-90.5, 5)
  line L29 (-90.5, 5) -> (-68.5, 5)
  line L30 (-68.5, 5) -> (-68.5, 35)
  line L31 (-68.5, 35) -> (-90.5, 5) construction
  line L32 (-90.5, 35) -> (-68.5, 5) construction
  point P0 (-54.5, 20)
  point P1 (-13, 20)
  point P2 (-79.5, 20)
  dimension "d175" = 20
  dimension "d176" = 10
  dimension "d177" = 27.5
  dimension "d178" = 20
  dimension "d179" = 7
  dimension "d180" = 4.5
  dimension "d181" = 7
  dimension "d182" = 3.5
  dimension "d183" = 8
  dimension "d184" = 8
  dimension "d185" = 8
  dimension "d186" = 8
  dimension "d241" = 25
  dimension "d242" = 22
  dimension "d243" = 30
  constraint horizontal L4
  constraint vertical L5
  constraint horizontal L6
  constraint vertical L7
  constraint coincident L0.end L1.start
  constraint horizontal L8
  constraint vertical L9
  constraint horizontal L10
  constraint vertical L11
  constraint midpoint L11 L12.start
  constraint perpendicular L11 L12
  constraint coincident P1 L12.end
  constraint midpoint L9 L13.start
  constraint perpendicular L9 L13
  constraint coincident P0 L13.end
  constraint horizontal L14
  constraint perpendicular L14 L15
  constraint parallel L14 L16
  constraint parallel L15 L17
  constraint coincident L18 P0
  constraint coincident L19 P0
  constraint horizontal L20
  constraint perpendicular L20 L21
  constraint parallel L20 L22
  constraint parallel L21 L23
  constraint coincident L24 P1
  constraint coincident L25 P1
  constraint parallel L13 L26
  constraint horizontal L27
  constraint perpendicular L27 L28
  constraint parallel L27 L29
  constraint parallel L28 L30
  constraint coincident L31 P2
  constraint coincident L32 P2
  constraint coincident P2 L26.end
  measures "d175" distance of L0.end L4.end
  measures "d176" distance of L0.end L6.end
  measures "d177" distance of L5.end L8.end
  measures "d178" distance of L5.end L10.end
  measures "d179" distance of L12.start P1
  measures "d180" diameter of A0
  measures "d181" distance of L13.start P0
  measures "d182" diameter of A1
  measures "d183" distance of L15.end L16.end
  measures "d184" distance of L14.end L15.end
  measures "d185" distance of L21.end L22.end
  measures "d186" distance of L20.end L21.end
  measures "d241" distance of P0 P2
  measures "d242" distance of L28.end L29.end
  measures "d243" distance of L27.end L28.end
extrude "Extrude26" cut sketch "Sketch19" against normal blind 6 contours L8 L9 L10 L11 | A0 | L13 A1 L26 | L13 A1 L26 | L27 L28 L29 L30 bodies 22
sketch "Sketch21" plane through (0, 0, 45) normal (0, 0, 1) x (-1, 0, 0)
  line L0 (-97, 11) -> (-97, 60)
  line L1 (-97, 60) -> (-100, 60)
  line L2 (-100, 60) -> (-100, 0)
  line L3 (-100, 0) -> (0, 0)
  line L4 (0, 0) -> (0, 60)
  line L5 (0, 60) -> (-3, 60)
  line L6 (-3, 60) -> (-3, 11)
  line L7 (-11, 3) -> (-89, 3)
  line L8 (0, 0) -> (-100, 0)
  line L9 (-100, 0) -> (-100, 60)
  line L10 (-100, 60) -> (0, 60)
  line L11 (0, 60) -> (0, 0)
  circle A0 centre (-93, 7) radius 1.6
  circle A1 centre (-7, 7) radius 1.6
  line L12 (-35, 61) -> (-65, 39) construction
  line L13 (-65, 61) -> (-35, 39) construction
  circle A2 centre (-93, 7) radius 2.25
  circle A3 centre (-7, 7) radius 2.25
  line L14 (-3, 11) -> (-11, 11)
  line L15 (-11, 11) -> (-11, 3)
  line L16 (-89, 3) -> (-89, 11)
  line L17 (-89, 11) -> (-97, 11)
  point P0 (-50, 50)
  dimension "d214" = 100
  dimension "d215" = 60
  dimension "d216" = 3.2
  dimension "d217" = 3.2
  dimension "d219" = 30
  dimension "d220" = 22
  constraint horizontal L8
  constraint vertical L9
  constraint horizontal L10
  constraint vertical L11
  constraint coincident L3.end L4.start
  constraint coincident L12 P0
  constraint coincident L13 P0
  constraint coincident A0.centre A2.centre
  measures "d214" distance of L3.end L2.end
  measures "d215" distance of L3.end L4.end
  measures "d216" diameter of A0
  measures "d217" diameter of A1
  measures "d219" distance of L12.end L13.end
  measures "d220" distance of L13.start L12.end
extrude "Extrude29" add sketch "Sketch21" along normal blind 3 separate body contours L0 L1 L2 L3 L4 L5 L6 L7 L8 L9 L10 L11 L14 L15 L16 L17 | L0 L6 L7 L10 L14 L15 L16 L17 | A2 | A3 makes body 27
extrude "Extrude30" add sketch "Sketch14" along normal blind 3 contours L3 L7 L17 L31 L32 L33 L34 | L4 L9 L13 L35 L36 L37 L38 bodies 22
extrude "Extrude35" add sketch "Sketch14" along normal blind 3 separate body contours L4 L42 L44 L45 L46 L47 | L42 L48 L49 L50 L51 makes body 28 at (4.9577, -64.1016, 0) makes body 29 at (95.0423, -64.1016, 0)
extrude "Extrude25" add sketch "Sketch19" against normal blind 6 contours L13 A1 L14 L15 L17 L26 | L13 A1 L15 L16 L17 L26 | L20 L21 L22 L23 bodies 22
chamfer "Chamfer9" distance 1.5 angle 45 4 edges at (106.585, -5.6147, 3) (-3.415, -5.6147, 3) (6.585, -68.6147, 3) (96.585, -68.6147, 3) on bodies 22 28 29
extrude "Extrude33" add sketch "Sketch14" along normal blind 48 separate body contours L4 L12 L16 L18 L19 L40 L41 L42 L43 L44 L48 makes body 30
combine "Combine3" operation add target body 27 tool bodies 30 29 28
move_body "Move4" bodies 22 27 to x (1, 0, 0) y (0, 1, 0) z (0, 0, 1) at (10, 0, 0)
sketch "Sketch22" plane through (0, -63, 0) normal (0, -1, 0) x (1, 0, 0)
  line L0 (20, 0) -> (100, 0)
  line L1 (110, 3) -> (110, 48)
  line L2 (110, 48) -> (10, 48)
  line L3 (10, 48) -> (10, 3)
  line L4 (100, 0) -> (85, 0)
  line L5 (85, 0) -> (65, 0)
  line L6 (65, 0) -> (65, 12)
  line L7 (65, 12) -> (85, 12)
  line L8 (85, 12) -> (85, 0)
  line L9 (20, 3) -> (20, 0)
  line L10 (100, 0) -> (100, 3)
  line L11 (100, 3) -> (110, 3)
  line L12 (10, 3) -> (20, 3)
  dimension "d248" = 15
  dimension "d249" = 20
  dimension "d250" = 12
  constraint coincident L0.end L4.start
  constraint perpendicular L1 L4
  constraint horizontal L5
  constraint vertical L6
  constraint horizontal L7
  constraint vertical L8
  measures "d248" distance of L0.end L4.end
  measures "d249" distance of L4.end L5.end
  measures "d250" distance of L4.end L7.end
extrude "Extrude34" cut sketch "Sketch22" against normal blind 3 contours L0 L5 L6 L7 L8 bodies 27
chamfer "Chamfer10" distance 5 angle 45 2 edges at (85, -61.5, 12) (65, -61.5, 12) on bodies 27
equation "d30 = ( 19 / 2 ) * 1 mm"
equation "d33 = ( 19 / 2 ) * 1 mm"
equation "d45 = 108.5 mm - 25 mm"
equation "d78 = ( -105 / 2 ) * 1 mm - 2 mm"
equation "d80 = ( 105 / 2 ) * 1 mm - 2 mm"
equation "d83 = ( 19 / 2 ) * 1 mm"
equation "d143 = 20.000 mm / 2"
equation "d144 = ( 19 / 2 ) * 1 mm"
equation "d149 = 147 mm - 22 mm"
named bodies: "Base", "MOT", "Top arm", "Bottom arm", "Bottom electrode", "Top electrode", "Spring", "DIN rail", "Bottom", "Top lug clip", "Bottom lug clip", "Bottom wire clip", "Top wire clip", "Top"
